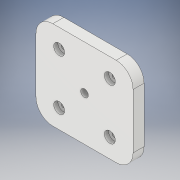
# Autodesk Inventor part: AA030
Saved by Autodesk Inventor 2017 SP1 (Build 210196100, 196)
## iProperties
Created: 2017-10-10
Part Number: AA030
Material: ABS Plastic
Document SubType Name: Modeling
Designer: Zach
Density: 1.06 g/cm^3
Appearance: CR White
Author: Zach
Autodesk Inventor part; units mm, degrees
ref_plane "YZ Plane" through (0, 0, 0) normal (1, 0, 0) x (0, 1, 0)
ref_plane "XZ Plane" through (0, 0, 0) normal (0, 1, 0) x (-1, 0, 0)
ref_plane "XY Plane" through (0, 0, 0) normal (0, 0, 1) x (1, 0, 0)
sketch "Sketch1" plane through (0, 0, 0) normal (0, 0, 1) x (1, 0, 0)
  line L0 (0, 0) -> (115, 0)
  line L1 (115, 0) -> (115, 105)
  line L2 (115, 105) -> (0, 105)
  line L3 (0, 105) -> (0, 0)
  circle A0 centre (57.5, 52.5) radius 4.5
  line L4 (27.5, 22.5) -> (87.5, 22.5) construction
  line L5 (87.5, 22.5) -> (87.5, 82.5) construction
  line L6 (87.5, 82.5) -> (27.5, 82.5) construction
  line L7 (27.5, 82.5) -> (27.5, 22.5) construction
  circle A1 centre (87.5, 82.5) radius 2.5
  circle A2 centre (27.5, 82.5) radius 2.5
  circle A3 centre (27.5, 22.5) radius 2.5
  circle A4 centre (87.5, 22.5) radius 2.5
  point P0 (57.5, 0)
  point P1 (0, 52.5)
  point P2 (27.5, 52.5)
  point P3 (57.5, 82.5)
  dimension "d0" = 115
  dimension "d1" = 105
  dimension "d2" = 9
  dimension "d3" = 60
  dimension "d4" = 60
  dimension "d5" = 5
  dimension "d6" = 5
  dimension "d7" = 5
  dimension "d8" = 5
  constraints: 16 end point, 5 centre point, 5 coincident, 4 midpoint, 4 parallel, 2 horizontal, 2 horizontal alignment, 2 perpendicular, 2 vertical alignment
  measures "d0" distance of L2.end L1.end
  measures "d1" distance of L1.end L0.end
  measures "d2" diameter of A0
  measures "d3" distance of L6.end L5.end
  measures "d4" distance of L5.end L4.end
  measures "d5" diameter of A1
  measures "d6" diameter of A2
  measures "d7" diameter of A3
  measures "d8" diameter of A4
extrude "Extrusion1" add sketch "Sketch1" along normal blind 13
fillet "Fillet1" radius 20 4 edges at (0, 105, 6.5) (115, 105, 6.5) (115, 0, 6.5) (0, 0, 6.5)
sketch "Sketch5" plane through (0, 0, 13) normal (0, 0, 1) x (1, 0, 0)
  circle A0 centre (27.5, 82.5) radius 2.5 projected
  circle A1 centre (87.5, 82.5) radius 2.5 projected
  circle A2 centre (87.5, 22.5) radius 2.5 projected
  circle A3 centre (27.5, 22.5) radius 2.5 projected
  circle A4 centre (87.5, 82.5) radius 6.5
  circle A5 centre (87.5, 22.5) radius 6.5
  circle A6 centre (27.5, 22.5) radius 6.5
  circle A7 centre (27.5, 82.5) radius 6.5
  point P0 (0, 0)
  dimension "d18" = 13
  dimension "d19" = 13
  dimension "d20" = 13
  dimension "d21" = 13
  constraints: 4 centre point, 4 coincident
  measures "d18" diameter of A4
  measures "d19" diameter of A5
  measures "d20" diameter of A6
  measures "d21" diameter of A7
extrude "Extrusion4" cut sketch "Sketch5" against normal blind 5 contours A0 | A1 | A2 | A3 | A4 | A5 | A6 | A7
body "Solid1"
